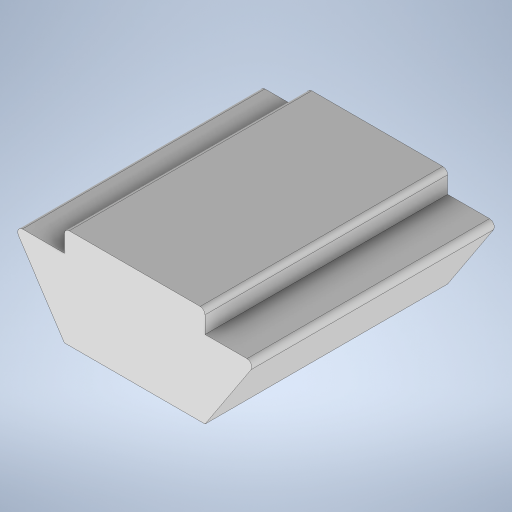
# Autodesk Inventor part: framespacer1
Saved by Autodesk Inventor 2024 (Build 280153000, 153)
## iProperties
Created: 2025-08-23
Part Number: framespacer1
Material: 一般
Document SubType Name: Modeling
Designer: tanoue_kota
Density: 1 g/cm^3
Appearance: 既定
Author: tanoue_kota
Autodesk Inventor part; units mm, degrees
ref_plane "YZ Plane" through (0, 0, 0) normal (1, 0, 0) x (0, 1, 0)
ref_plane "XZ Plane" through (0, 0, 0) normal (0, 1, 0) x (-1, 0, 0)
ref_plane "XY Plane" through (0, 0, 0) normal (0, 0, 1) x (1, 0, 0)
sketch "スケッチ1" plane through (0, 0, 0) normal (0, 0, 1) x (1, 0, 0)
  line L0 (0, 0) -> (2.9, 0)
  line L1 (2.9, 0) -> (5, 3.2)
  line L2 (5, 3.2) -> (0, 3.2)
  line L3 (0, 0) -> (0, 4)
  line L4 (0, 3.2) -> (2.9, 3.2)
  line L5 (2.9, 3.2) -> (2.9, 4.1)
  line L6 (2.9, 4.1) -> (0, 4.1)
  line L7 (0, 4.1) -> (0, 3.2)
  line L8 (0, 0) -> (-2.9, 0)
  line L9 (-2.9, 0) -> (-5, 3.2)
  line L10 (-5, 3.2) -> (0, 3.2)
  line L11 (-2.9, 3.2) -> (-2.9, 4.1)
  line L12 (-2.9, 4.1) -> (0, 4.1)
  dimension "d0" = 3.2
  dimension "d1" = 5
  dimension "d2" = 2.9
  dimension "d3" = 2.9
  dimension "d4" = 4.1
  constraints: 26 end point, 4 symmetric about line, 3 parallel, 2 horizontal, 1 perpendicular, 1 point on line, 1 vertical
  measures "d0" distance between parallel lines of L0 L2
  measures "d1" distance of L1.end L2.end
  measures "d2" distance of L0.start L0.end
  measures "d3" distance of L5.end L6.end
  measures "d4" distance between parallel lines of L0 L6
extrude "押し出し1" add sketch "スケッチ1" along normal blind 10
fillet "フィレット1" radius 0.2 2 edges at (5, 3.2, 5) (-5, 3.2, 5)
fillet "フィレット2" radius 0.2 2 edges at (-2.9, 4.1, 5) (2.9, 4.1, 5)
